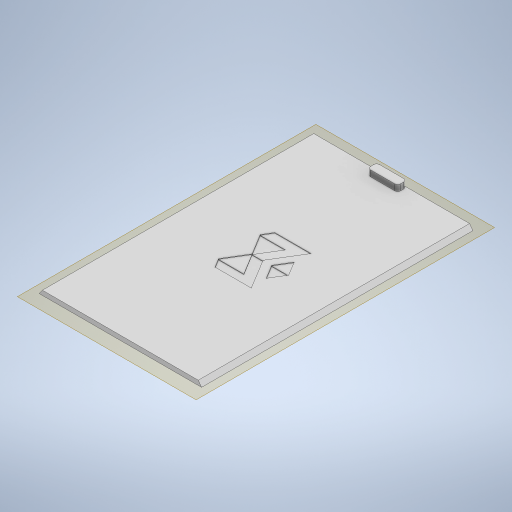
# Autodesk Inventor part: cover2
Saved by Autodesk Inventor 2023 (Build 270158000, 158)
## iProperties
Created: 2023-03-10
Part Number: cover2
Material: Типовые
Document SubType Name: Modeling
Designer: Josh
Density: 1 g/cm^3
Appearance: По умолчанию
Author: Josh
Autodesk Inventor part; units mm, degrees
ref_plane "YZ Plane" through (0, 0, 0) normal (1, 0, 0) x (0, 1, 0)
ref_plane "XY Plane" through (0, 0, 0) normal (0, 0, 1) x (1, 0, 0)
sketch "Эскиз1" plane through (0, 0, 0) normal (0, 0, 1) x (1, 0, 0)
  line L0 (0, -0.6) -> (0, 3.6) projected
  line L1 (0, 0) -> (0, 3)
  line L2 (-24.75, 3) -> (24.75, 3)
  line L3 (-26.95, 0) -> (26.95, 0)
  line L4 (-24.75, 3) -> (-26.95, 0)
  line L5 (24.75, 3) -> (26.95, 0)
  line L6 (-25.85, 1.5) -> (25.85, 1.5)
  dimension "d1" = 3
  dimension "d3" = 49.5
  dimension "d4" = 53.9
  constraints: 12 end point, 4 midpoint, 2 horizontal, 1 point on line
  measures "d1" distance of L1.end L1.start
  measures "d3" distance of L2.start L2.end
  measures "d4" distance of L3.start L3.end
extrude "Выдавливание1" add sketch "Эскиз1" along normal blind 90 contours L3 L4 L6 L0 | L0 L6 L5 L3
sketch "Эскиз2" plane through (-25.85, 1.5, 0) normal (0, 1, 0) x (1, 0, 0)
  line L0 (-1.1, 0) -> (52.8, 0) projected
  line L1 (20.85, 0) -> (30.85, 0)
  line L2 (30.85, 0) -> (30.85, -3)
  line L3 (30.85, -3) -> (20.85, -3)
  line L4 (20.85, -3) -> (20.85, 0)
  line L5 (25.85, 18) -> (25.85, -108) projected
  point P0 (25.85, 0)
  dimension "d7" = 10
  dimension "d8" = 3
  constraints: 8 end point, 2 parallel, 1 horizontal, 1 perpendicular, 1 point on line, 1 other
  measures "d7" distance between parallel lines of L2 L4
  measures "d8" distance between parallel lines of L0 L3
extrude "Выдавливание2" add sketch "Эскиз2" along normal blind 2
fillet "Сопряжение1" radius 1 4 edges at (5, 2.5, 3) (5, 2.5, 0) (-5, 2.5, 3) (-5, 2.5, 0)
sketch "Эскиз7" plane through (-25.85, 1.5, 90) normal (0, 1, 0) x (1, 0, 0)
  line L0 (0, 90) -> (-1.1, 90) projected
  line L1 (45.7625, 90) -> (45.7625, 0) construction
  line L2 (45.7625, 0) -> (5.9375, 0) construction
  line L3 (5.9375, 0) -> (5.9375, 90) construction
  line L4 (5.9375, 90) -> (45.7625, 90) construction
  line L5 (51.7, 0) -> (0, 0) projected
  line L6 (-1.1, 0) -> (52.8, 0) projected
  line L7 (21.9773, 55.1118) -> (20.1462, 52.0958)
  line L8 (20.1462, 52.0958) -> (24.3419, 45.1851)
  line L9 (21.9773, 55.1118) -> (34.0311, 55.1118)
  line L10 (34.0311, 55.1118) -> (28.0042, 45.1851)
  line L11 (28.0042, 45.1851) -> (24.3419, 45.1851)
  line L12 (20.1462, 52.0958) -> (28.5377, 52.0958)
  line L13 (28.5377, 52.0958) -> (24.3419, 45.1851)
  line L14 (30.8592, 45.1851) -> (36.522, 45.1851)
  line L15 (36.522, 45.1851) -> (33.6906, 49.8437)
  line L16 (33.6906, 49.8437) -> (30.8592, 45.1851)
  line L17 (33.6906, 49.8437) -> (33.6906, 45.1851) construction
  line L18 (24.3419, 45.1851) -> (24.3419, 52.0958) construction
  line L19 (28.0042, 45.1851) -> (28.0042, 55.1118) construction
  line L20 (21.9773, 35.2585) -> (20.1462, 38.2745)
  line L21 (20.1462, 38.2745) -> (24.3419, 45.1851)
  line L22 (21.9773, 35.2585) -> (34.0311, 35.2585)
  line L23 (34.0311, 35.2585) -> (28.0042, 45.1851)
  line L24 (20.1462, 38.2745) -> (28.5377, 38.2745)
  line L25 (28.5377, 38.2745) -> (24.3419, 45.1851)
  line L26 (36.522, 45.1851) -> (33.6906, 40.5265)
  line L27 (33.6906, 40.5265) -> (30.8592, 45.1851)
  line L28 (33.6906, 40.5265) -> (33.6906, 45.1851) construction
  line L29 (24.3419, 45.1851) -> (24.3419, 38.2745) construction
  line L30 (28.0042, 45.1851) -> (28.0042, 35.2585) construction
  point P0 (25.85, 90)
  point P1 (51.7, 90)
  point P2 (25.85, 0)
  constraints: 50 end point, 10 symmetric about line, 6 midpoint, 3 parallel, 3 point on line, 2 horizontal, 2 perpendicular, 1 vertical, 1 vertical alignment, 2 other
emboss "Рельеф1" sketch "Эскиз7" operation cut depth 0.4 direction (0, -1, 0) contours L12 L13 L8 | L11 L23 L22 L20 L24 L25 | L14 L26 L27
sketch "Эскиз8" plane through (-25.85, 1.5, 90) normal (0, 1, 0) x (1, 0, 0)
  line L0 (30.8592, 45.1851) -> (36.522, 45.1851) projected
  line L1 (33.6906, 40.5265) -> (30.8592, 45.1851) projected
  line L2 (36.522, 45.1851) -> (33.6906, 40.5265) projected
  line L3 (24.3419, 45.1851) -> (28.0042, 45.1851) projected
  line L4 (28.5377, 38.2745) -> (24.3419, 45.1851) projected
  line L5 (20.1462, 38.2745) -> (28.5377, 38.2745) projected
  line L6 (21.9773, 35.2585) -> (20.1462, 38.2745) projected
  line L7 (34.0311, 35.2585) -> (21.9773, 35.2585) projected
  line L8 (28.0042, 45.1851) -> (34.0311, 35.2585) projected
  line L9 (20.1462, 52.0958) -> (28.5377, 52.0958) projected
  line L10 (24.3419, 45.1851) -> (20.1462, 52.0958) projected
  line L11 (28.5377, 52.0958) -> (24.3419, 45.1851) projected
  line L12 (33.6906, 49.8437) -> (30.8592, 45.1851)
  line L13 (36.522, 45.1851) -> (33.6906, 49.8437)
  line L14 (28.5377, 52.0958) -> (24.3419, 45.1851)
  line L15 (20.1462, 52.0958) -> (28.5377, 52.0958)
  line L16 (21.9773, 55.1118) -> (20.1462, 52.0958)
  line L17 (34.0311, 55.1118) -> (21.9773, 55.1118)
  line L18 (28.0042, 45.1851) -> (34.0311, 55.1118)
  line L19 (20.1462, 38.2745) -> (28.5377, 38.2745)
  line L20 (24.3419, 45.1851) -> (20.1462, 38.2745)
  line L21 (28.5377, 38.2745) -> (24.3419, 45.1851)
  point P0 (25.85, 90)
  constraints: 20 end point, 7 symmetric about line
extrude "Выдавливание3" cut sketch "Эскиз8" against normal blind 0.2 contours L12 L13 L0 | L11 L9 L16 L17 L18 L3 | L4 L5 L20
